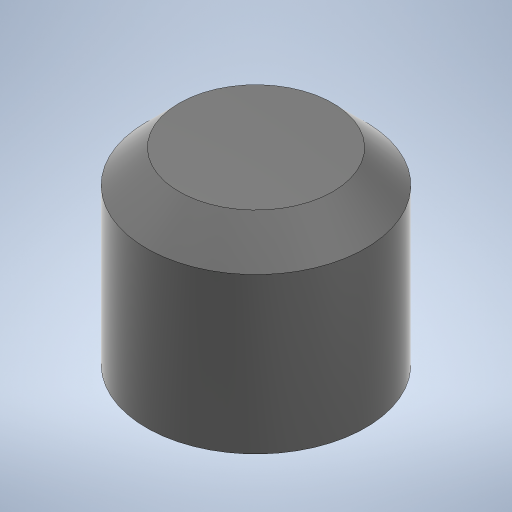
# Autodesk Inventor part: AeroSky_MC4230-630KV
Saved by Autodesk Inventor 2023 (Build 270158000, 158)
## iProperties
Created: 2022-07-20
Part Number: AeroSky_MC4230-630KV
Material: Stainless Steel, Austenitic
Document SubType Name: Modeling
Designer: Nathan Cai
Density: 2.83653 g/cm^3
Appearance: Smooth - Black
Mass: 140 g
Surface Area: 71.6152 cm^2
Volume: 49.3561 cm^3
Author: Nathan Cai
Autodesk Inventor part; units mm, degrees
ref_plane "YZ Plane" through (0, 0, 0) normal (1, 0, 0) x (0, 1, 0)
ref_plane "XZ Plane" through (0, 0, 0) normal (0, 1, 0) x (-1, 0, 0)
ref_plane "XY Plane" through (0, 0, 0) normal (0, 0, 1) x (1, 0, 0)
sketch "Sketch1" plane through (0, 0, 0) normal (0, 1, 0) x (-1, 0, 0)
  circle A0 centre (0, 0) radius 21.25
  dimension "d0" = 42.5
  constraints: 1 centre point, 1 coincident
  measures "d0" diameter of A0
extrude "Extrusion1" add sketch "Sketch1" along normal blind 36.5
chamfer "Chamfer1" distance 6.35 angle 45 1 edges at (21.25, 36.5, 0)
body "Solid1"
